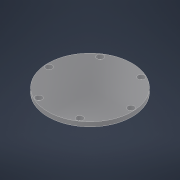
# Autodesk Inventor part: P021-Bouchon_carter_vilbrequin
Saved by Autodesk Inventor 2021.3 (Build 253353000, 353)
## iProperties
Created: 2022-06-06
Part Number: P021-Bouchon_carter_vilbrequin
Material: Aluminium
Document SubType Name: Modeling
Designer: Rémi Heredero
Density: 2.7 g/cm^3
Appearance: Aluminum - Dark
Author: Rémi Heredero
Autodesk Inventor part; units mm, degrees
ref_plane "YZ Plane" through (0, 0, 0) normal (1, 0, 0) x (0, 1, 0)
ref_plane "XZ Plane" through (0, 0, 0) normal (0, 1, 0) x (-1, 0, 0)
ref_plane "XY Plane" through (0, 0, 0) normal (0, 0, 1) x (1, 0, 0)
sketch "Sketch2" plane through (0, 0, 0) normal (0, 0, 1) x (1, 0, 0)
  circle A0 centre (0, 0) radius 30
  dimension "d0" = 60
  constraints: 1 centre point, 1 coincident
  measures "d0" diameter of A0
extrude "Extrusion1" add sketch "Sketch2" along normal blind 3
sketch "Sketch5" plane through (0, 0, 0) normal (0, 0, -1) x (-1, 0, 0)
  circle A0 centre (-11.6503, 24.0797) radius 1.621 construction
  circle A1 centre (-15.0285, -22.1293) radius 1.621 construction
  circle A2 centre (26.6788, -1.9504) radius 1.621 construction
  circle A3 centre (11.6503, -24.0797) radius 1.621 construction
  circle A4 centre (-26.6788, 1.9504) radius 1.621 construction
  circle A5 centre (15.0285, 22.1293) radius 1.621 construction
  circle A6 centre (0, 0) radius 23.5 construction
  line L0 (49.4604, 10.5316) -> (7.3244, -51.5131) construction
  line L1 (-8.448, 49.8586) -> (49.4604, 10.5316) construction
  line L2 (-50.5841, -12.1861) -> (-8.448, 49.8586) construction
  line L3 (7.3244, -51.5131) -> (-50.5841, -12.1861) construction
  point P0 (0, 0)
hole "Hole2" at (-15.0285, 22.1293, 0) at (-26.6788, -1.9504, 0) at (-11.6503, -24.0797, 0) at (15.0285, -22.1293, 0) at (26.6788, 1.9504, 0) at (11.6503, 24.0797, 0) direction (0, 0, 1) diameter 4.5 end through all start extended yes clearance for "Countersunk Flat Head Screw ISO 2009/7046" size "M4" standard "ISO"
body "Solid1"
